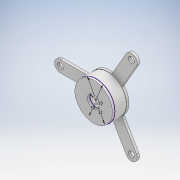
# Autodesk Inventor part: Pok Mk3 Yaw Motor Mount Mk2
Saved by Autodesk Inventor 2018.2 (Build 222227000, 227)
## iProperties
Created: 2018-02-27
Part Number: Pok Mk3 Yaw Motor Mount Mk2
Material: ABS Plastic
Document SubType Name: Modeling
Designer: Moochster
Density: 1.06 g/cm^3
Appearance: Smooth - White
Author: Moochster
Autodesk Inventor part; units mm, degrees
ref_plane "YZ Plane" through (0, 0, 0) normal (1, 0, 0) x (0, 1, 0)
ref_plane "XZ Plane" through (0, 0, 0) normal (0, 1, 0) x (-1, 0, 0)
ref_plane "XY Plane" through (0, 0, 0) normal (0, 0, 1) x (1, 0, 0)
sketch "Sketch1" plane through (0, 0, 0) normal (0, 1, 0) x (-1, 0, 0)
  circle A0 centre (0, 0) radius 15
  circle A1 centre (0, 0) radius 16.2
  line L0 (15.4091, 5) -> (40.4091, 5)
  arc A2 (40.4091, -5) -> (40.4091, 5) centre (40.4091, 0) ccw
  line L1 (40.4091, -5) -> (15.4091, -5)
  circle A3 centre (40.4091, 0) radius 2.5
  dimension "d0" = 30
  dimension "d1" = 1.2
  dimension "d2" = 5
  dimension "d3" = 25
  dimension "d4" = 5
  constraints: 4 centre point, 4 end point, 4 point on circle, 3 coincident, 2 tangent, 1 horizontal, 1 horizontal alignment, 1 parallel
  measures "d0" diameter of A0
  measures "d1" radial gap between concentric circles of A0 A1
  measures "d2" distance from line of A2.centre L1
  measures "d3" distance of L1.start L1.end
  measures "d4" diameter of A3
extrude "Extrusion1" add sketch "Sketch1" along normal blind 2 contours A1 L0 A2 L1
extrude "Extrusion2" add sketch "Sketch1" along normal blind 2 contours A1
ref_plane "Work Plane1" through (0, -10, 0) normal (0, -1, 0) x (1, 0, 0)
sketch "Sketch2" plane through (0, -10, 0) normal (0, -1, 0) x (1, 0, 0)
  circle A0 centre (0, 0) radius 5.25
  circle A1 centre (0, 0) radius 16
  circle A2 centre (0, 0) radius 15
  dimension "d10" = 10.5
  dimension "d11" = 32
  dimension "d12" = 30
  constraints: 3 centre point, 3 coincident
  measures "d10" diameter of A0
  measures "d11" diameter of A1
  measures "d12" diameter of A2
extrude "Extrusion3" add sketch "Sketch2" along normal blind 2 contours A1 | A2
extrude "Extrusion4" add sketch "Sketch2" against normal up to surface (10 mm away) contours A1
pattern_circular "Circular Pattern1" count 3 over 360 about axis through (0, -10, 0) along (0, -1, 0) of "Extrusion1"
body "Solid1"
